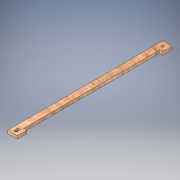
# Autodesk Inventor part: Wood Rail
Saved by Autodesk Inventor 2018 (Build 220112000, 112)
## iProperties
Created: 2017-12-04
Part Number: Wood Rail
Material: Generic
Document SubType Name: Modeling
Designer: Andrew
Density: 1 g/cm^3
Appearance: Birch - Natural Polished
d0: 0.125 in
d1: 0.375 in
d2: 0.375 in
d3: 6.125 in
d4: 0.100 in
d5: 0.056 in
d6: 0.125 in
d7: 0.00 deg
d10: 0.112 in
woodThickness: 0.125 in
Author: Andrew
Autodesk Inventor part; units mm, degrees
ref_plane "YZ Plane" through (0, 0, 0) normal (1, 0, 0) x (0, 1, 0)
ref_plane "XZ Plane" through (0, 0, 0) normal (0, 1, 0) x (-1, 0, 0)
ref_plane "XY Plane" through (0, 0, 0) normal (0, 0, 1) x (1, 0, 0)
sketch "Sketch1" plane through (0, 0, 0) normal (0, 1, 0) x (-1, 0, 0)
  line L0 (0, 68.2625) -> (3.175, 68.2625)
  line L1 (3.175, 68.2625) -> (3.175, -68.2625)
  line L2 (3.175, -68.2625) -> (0, -68.2625)
  line L3 (0, -68.2625) -> (0, -77.7875)
  line L4 (0, -77.7875) -> (9.525, -77.7875)
  line L5 (9.525, -77.7875) -> (9.525, 77.7875)
  line L6 (9.525, 77.7875) -> (0, 77.7875)
  line L7 (0, 77.7875) -> (0, 68.2625)
  line L8 (-1.905, 0) -> (11.43, 0) construction
  line L9 (4.7625, 74.295) -> (4.7625, 71.755) construction
  line L10 (3.3401, 74.295) -> (3.3401, 71.755)
  line L11 (6.1849, 71.755) -> (6.1849, 74.295)
  arc A0 (6.1849, 74.295) -> (3.3401, 74.295) centre (4.7625, 74.295) ccw
  arc A1 (3.3401, 71.755) -> (6.1849, 71.755) centre (4.7625, 71.755) ccw
  circle A2 centre (4.7625, -73.025) radius 1.4224
  point P0 (0, 0)
  point P1 (4.7625, 73.025)
  point P2 (0, 73.025)
  point P3 (0, -73.025)
  point P4 (4.7625, -77.7875)
  point P5 (4.7625, 77.7875)
  dimension "d0" = 3.175
  dimension "d1" = 9.525
  dimension "d2" = 9.525
  dimension "d3" = 155.575
  dimension "d4" = 2.54
  dimension "d5" = 1.4224
  dimension "d10" = 2.8448
  constraints: 24 end point, 7 perpendicular, 5 midpoint, 4 point on circle, 4 tangent, 3 centre point, 2 horizontal alignment, 2 point on line, 2 vertical alignment, 1 horizontal, 1 parallel, 1 vertical, 2 other
  measures "d0" distance of L0.start L0.end
  measures "d1" distance of L5.end L6.end
  measures "d2" distance of L6.end L0.start
  measures "d3" distance between parallel lines of L4 L6
  measures "d4" distance of L9.start L9.end
  measures "d5" radius of A0
  measures "d10" diameter of A2
extrude "Extrusion1" add sketch "Sketch1" along normal mid plane 3.175
equation "\"d10\" = 2 * d5"
equation "\"woodThickness\" = 3.175"
body "Solid1"
